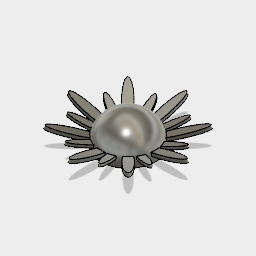
FPROJ_5 (Autodesk Fusion 360 design; units mm, degrees)
Autodesk Fusion 360 part; units mm, degrees
sketch "草图1" plane through (0, 0, 0) normal (0, 0, 1) x (1, 0, 0)
  ellipse E0 centre (0, 0) end of major axis (20, 0) minor radius 4
  line L0 (-20, 0) -> (20, 0)
  line L1 (0, -4) -> (0, 4)
extrude "拉伸1" add sketch "草图1" along normal blind 3 makes body 1
move_body "移动1" bodies 1 to x (1, 0, 0) y (0, 0, 1) z (0, -1, 0) at (0, -4, 4)
move_body "移动2" bodies 1 to x (0.965926, 0.258819, 0) y (-0.258819, 0.965926, 0) z (0, 0, 1) at (33.7013, 4.9379, -4.1197)
move_body "移动3" bodies 1 to x (1, 0, 0) y (0, 1, 0) z (0, 0, 1) at (-15.8903, 6.7681, 0)
move_body "移动4" bodies 1 to x (1, 0, 0) y (0, 1, 0) z (0, 0, 1) at (14.7132, 0.5885, 0)
pattern_circular "C-阵列1" count 8 over 360 about axis through (0, 1.75, 0) along (0, 1, 0) of bodies 1 makes body 2 at (21.4189, 6.5881, -27.2442) makes body 3 at (-4.1192, 7.5449, -34.1173) makes body 4 at (-27.2442, 6.5881, -21.4189) makes body 5 at (-37.4084, 7.3915, 4.0598) makes body 6 at (-23.4243, 8.367, 29.1638) makes body 7 at (4.0598, 7.3915, 37.4084) makes body 8 at (27.2442, 6.5881, 21.4189)
copy_body "复制和粘贴实体1" bodies 8 2 3 7 4 5 1 6 makes body 9 makes body 10 makes body 11 makes body 12 makes body 13 makes body 14 makes body 15 makes body 16
move_body "移动5" bodies 9 10 11 12 13 14 15 16 to x (1, 0, 0) y (0, 1, 0) z (0, 0, 1) at (82.7017, -9.2188, 0.6474)
scale "缩放1" factor 0.8 about (93.236, -8.8622, -10.0562) bodies 12 13 14 15 16 9 11 10
move_body "移动6" bodies 11 12 13 14 15 16 10 9 to x (0.906308, 0, 0.422618) y (0, 1, 0) z (-0.422618, 0, 0.906308) at (-11.1343, 0, -38.6103)
move_body "移动7" bodies 9 12 16 15 13 14 11 10 to x (1, 0, 0) y (0, 1, 0) z (0, 0, 1) at (-66.5832, 0, 4.3083)
move_body "移动8" bodies 14 9 13 10 15 16 12 11 to x (1, 0, 0) y (0, 1, 0) z (0, 0, 1) at (0, 8.9232, -0.1352)
sphere "球体基本要素1" add diameter 50 placed x (1, 0, 0) y (0, 0, -1) z (0, 1, 0) at (0, 0, 0) bodies 1 2 3 4 5 6 7 8 9 10 11 12 13 14 15 16
box "长方体基本要素1" add length 200 width 200 height 50 placed x (0, 0, 1) y (1, 0, 0) z (0, 1, 0) at (0, 0, 0) separate body makes body 17
move_body "移动9" bodies 17 to x (1, 0, 0) y (0, 1, 0) z (0, 0, 1) at (-100.4055, 0, -109.2067)
move_body "移动10" bodies 1 to x (1, 0, 0) y (0, 1, 0) z (0, 0, 1) at (0.5618, 36.2368, 0)
move_body "移动11" bodies 1 to x (1, 0, 0) y (0, 1, 0) z (0, 0, 1) at (0, 30.6184, 0)
move_body "移动12" bodies 1 to x (1, 0, 0) y (0, 1, 0) z (0, 0, 1) at (0, -14.0459, 0)
combine "合并1" operation cut target body 1 tool bodies 17
